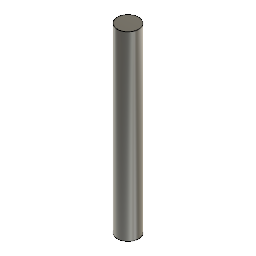
Wheel hub nut dowel pin (Autodesk Fusion 360 design; units mm, degrees)
Autodesk Fusion 360 part; units mm, degrees
sketch "Sketch1" plane through (0, 0, 0) normal (0, 0, 1) x (1, 0, 0)
  circle A0 centre (0, 0) radius 1.65
  dimension "d4" = 3.3
  constraint coincident A0.centre origin
  measures "d4" diameter of A0
extrude "Extrude1" add sketch "Sketch1" along normal blind 28
equation "dowel_pin_radius = 1.65 mm"
equation "length = 28 mm"
equation "d4 = dowel_pin_radius * 2"
equation "d5 = length"
